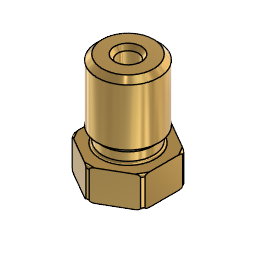
V6 0.4mm Nozzle (No Threads) (Autodesk Fusion 360 design; units mm, degrees)
Autodesk Fusion 360 part; units mm, degrees
note: some values were not read from the file. Set by a fixed rule: which sketch regions a step uses.
sketch "Sketch1" plane through (0, 0, 0) normal (0, 1, 0) x (1, 0, 0)
  line L0 (-0.5, 0) -> (0.5, 0)
  line L1 (-0.2, 0) -> (-0.2, -0.6)
  line L2 (-0.2, -0.6) -> (-1, -1.9856)
  line L3 (-1, -1.9856) -> (-1, -12.0716)
  line L4 (-4.4259, -12.5) -> (0, -12.5)
  line L5 (0, -12.5) -> (0, 0)
  line L6 (-1, -12.0716) -> (-1.3, -12.5)
  line L7 (-1.3, -12.5) -> (-4.4259, -12.5)
  line L8 (-0.5, 0) -> (-1.8407, -1.9147)
  arc A0 (-0.3959, 0) -> (-0.5597, -0.0853) centre (-0.3959, -0.2) ccw
  line L9 (-2.0045, -2) -> (-3.5, -2)
  line L10 (-3.5, -2) -> (-3.5, -5)
  line L11 (-3.5, -5) -> (-2.7, -5)
  line L12 (-2.5, -5.2) -> (-2.5, -6)
  line L13 (-2.5, -6) -> (-3, -6.5)
  line L14 (-3, -6.5) -> (-3, -12)
  line L15 (-3, -12) -> (-2.5, -12.5)
  arc A1 (-2.0045, -2) -> (-1.8407, -1.9147) centre (-2.0045, -1.8) ccw
  arc A2 (-2.5, -5.2) -> (-2.7, -5) centre (-2.7, -5.2) ccw
  point P0 (-1.9004, -2)
  dimension "d3" = 0.2
  dimension "d5" = 30
  dimension "d10" = 12.5
  dimension "d11" = 1.3
  dimension "d12" = 1
  dimension "d14" = 125
  dimension "d15" = 0.6
  dimension "d16" = 1
  dimension "d17" = 0.2
  dimension "d18" = 2
  dimension "d19" = 3.5
  dimension "d20" = 5
  dimension "d21" = 2.5
  dimension "d24" = 3
  dimension "d25" = 135
  dimension "d26" = 135
  dimension "d27" = 0.5
  dimension "d28" = 1
  dimension "d29" = 0.2
  dimension "d38" = 0.2
  constraint horizontal L0
  constraint midpoint L5.end L0
  constraint coincident L0 L1.start
  constraint perpendicular L0 L1
  constraint perpendicular L0 L3
  constraint perpendicular L3 L4
  constraint coincident L5.end origin
  constraint vertical L5
  constraint parallel L4 L7
  constraint tangent L0 A0
  constraint coincident L0 A0.start
  constraint coincident L8 A0.end
  constraint tangent L8 A0
  constraint parallel L6 L8
  constraint horizontal L9
  constraint perpendicular L9 L10
  constraint perpendicular L10 L11
  constraint perpendicular L11 L12
  constraint parallel L12 L14
  constraint coincident L4 L15.end
  constraint coincident P0 L8
  constraint coincident P0 L9
  constraint tangent L8 A1
  constraint tangent L9 A1
  constraint tangent L12 A2
  constraint tangent L11 A2
  measures "d3" distance of L1 L5
  measures "d5" angle of L2 L5
  measures "d10" distance of L0 L4
  measures "d11" distance of L4.end L6.end
  measures "d12" distance of L3 L5
  measures "d14" angle of L4 L6
  measures "d15" distance of L1.start L1.end
  measures "d16" distance of L0.start L0.end
  measures "d17" radius of A0
  measures "d18" distance of L0 P0
  measures "d19" distance of L5 L10
  measures "d20" distance of L0 L11
  measures "d21" distance of L5 L12
  measures "d24" distance of L5 L14
  measures "d25" angle of L12 L13
  measures "d26" angle of L14 L15
  measures "d27" vertical distance of L14.end L15.end
  measures "d28" distance of L11 L12.end
  measures "d29" radius of A1
  measures "d38" radius of A2
revolve "Revolve1" add sketch "Sketch1" angle 360 about axis through (0, 0, 12.5) along (0, 0, -1) contours L0 L1 L2 L3 L4 L6 L7 L8 A0 L9 L10 L11 L12 L13 L14 L15 A1 A2
sketch "Sketch2" plane through (0, 0, 2) normal (0, 0, -1) x (1, 0, 0)
  circle A0 centre (0, 0) radius 3.5
  circle A1 centre (0, 0) radius 2.0045
  line L0 (-3.5, -2.0207) -> (0, -4.0415)
  line L1 (0, -4.0415) -> (3.5, -2.0207)
  line L2 (3.5, -2.0207) -> (3.5, 2.0207)
  line L3 (3.5, 2.0207) -> (0, 4.0415)
  line L4 (0, 4.0415) -> (-3.5, 2.0207)
  line L5 (-3.5, 2.0207) -> (-3.5, -2.0207)
  line L6 (-0.1584, 3.95) -> (0.1584, 3.95)
  line L7 (-0.1584, -3.95) -> (0.1584, -3.95)
  line L8 (0, 3.95) -> (0, -3.95) construction
  line L9 (-3.3416, -2.1122) -> (-3.5, -1.8378)
  line L10 (3.5, 1.8378) -> (3.3416, 2.1122)
  line L11 (3.5, -1.8378) -> (3.3416, -2.1122)
  line L12 (-3.3416, 2.1122) -> (-3.5, 1.8378)
  dimension "d31" = 7.9
  dimension "d33" = 360
  constraint coincident A0.centre A1.centre
  constraint vertical L5
  constraint tangent A0 L5
  constraint coincident L4 L6.start
  constraint coincident L3 L6.end
  constraint horizontal L6
  constraint coincident L0 L7.start
  constraint coincident L1 L7.end
  constraint parallel L6 L7
  constraint midpoint L6 L8.start
  constraint midpoint L7 L8.end
  constraint midpoint A0.centre L8
  measures "d31" distance of L6 L7
extrude "Extrude1" add sketch "Sketch2" against normal up to surface (3 mm away) contours A0 L1 L2 L11 | A0 L2 L3 L10 | A0 L3 L4 L6 | A0 L0 L1 L7 | A0 L4 L5 L12 | A0 L0 L5 L9
fillet "Fillet1" radius 0.2 12 edges at (3.4208, -1.975, 2) (3.4208, -1.975, 5) (0, -3.95, 5) (0, -3.95, 2) (-3.4208, -1.975, 2) (-3.4208, -1.975, 5) (-3.4208, 1.975, 5) (-3.4208, 1.975, 2) (0, 3.95, 5) (0, 3.95, 2) (3.4208, 1.975, 2) (3.4208, 1.975, 5)
equation "Table_D = 2 mm"
equation "d3 = Nozzle_Diameter / 2"
equation "Nozzle_Diameter = 0.4 mm"
equation "Table_C = 0.6 mm"
equation "Table_B = 1 mm"
equation "Table_F = 0.2 mm"
equation "Table_E = 2.6 mm"
equation "d11 = Table_E / 2"
equation "d12 = Table_D / 2"
equation "d15 = Table_C"
equation "d16 = Table_B"
equation "d17 = Table_F"
equation "d26 = d25"
equation "d29 = Table_F"
equation "d37 = Table_F"
